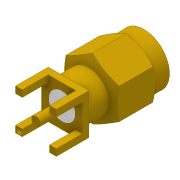
# Autodesk Inventor part: PE4525
Saved by Autodesk Inventor 2017 (Build 210142000, 142)
## iProperties
Created: 2020-05-17
Part Number: PE4525
Material: Aluminum 6061
Document SubType Name: Modeling
Designer: Flash
Density: 2.7 g/cm^3
Appearance: Gold
Author: Flash
Autodesk Inventor part; units mm, degrees
ref_plane "YZ Plane" through (0, 0, 0) normal (1, 0, 0) x (0, 1, 0)
ref_plane "XZ Plane" through (0, 0, 0) normal (0, 1, 0) x (-1, 0, 0)
ref_plane "XY Plane" through (0, 0, 0) normal (0, 0, 1) x (1, 0, 0)
sketch "Sketch1" plane through (0, 0, 0) normal (0, 1, 0) x (-1, 0, 0)
  line L0 (3.05, 3.05) -> (2.05, 3.05)
  line L1 (2.05, 3.05) -> (2.05, 2.05)
  line L2 (2.05, 2.05) -> (3.05, 2.05)
  line L3 (3.05, 2.05) -> (3.05, 3.05)
  line L4 (3.05, 3.05) -> (2.05, 2.05) construction
  line L5 (2.05, 3.05) -> (3.05, 2.05) construction
  line L6 (3.05, -3.05) -> (2.05, -3.05)
  line L7 (2.05, -3.05) -> (2.05, -2.05)
  line L8 (2.05, -2.05) -> (3.05, -2.05)
  line L9 (3.05, -2.05) -> (3.05, -3.05)
  line L10 (3.05, -3.05) -> (2.05, -2.05) construction
  line L11 (2.05, -3.05) -> (3.05, -2.05) construction
  line L12 (-2.05, -2.05) -> (-3.05, -2.05)
  line L13 (-3.05, -2.05) -> (-3.05, -3.05)
  line L14 (-3.05, -3.05) -> (-2.05, -3.05)
  line L15 (-2.05, -3.05) -> (-2.05, -2.05)
  line L16 (-2.05, -2.05) -> (-3.05, -3.05) construction
  line L17 (-3.05, -2.05) -> (-2.05, -3.05) construction
  line L18 (-2.05, 3.05) -> (-3.05, 3.05)
  line L19 (-3.05, 3.05) -> (-3.05, 2.05)
  line L20 (-3.05, 2.05) -> (-2.05, 2.05)
  line L21 (-2.05, 2.05) -> (-2.05, 3.05)
  line L22 (-2.05, 3.05) -> (-3.05, 2.05) construction
  line L23 (-3.05, 3.05) -> (-2.05, 2.05) construction
  line L24 (0, 0) -> (1.0097, 0)
  line L25 (1.0097, 0) -> (0, 0)
  line L26 (0, 0) -> (0, -1.0471)
  circle A0 centre (0, 0) radius 0.65
  point P0 (2.55, 2.55)
  point P1 (2.55, -2.55)
  point P2 (-2.55, -2.55)
  point P3 (-2.55, 2.55)
  dimension "d0" = 1
  dimension "d1" = 1
  dimension "d2" = 1
  dimension "d3" = 1
  dimension "d4" = 1
  dimension "d5" = 1
  dimension "d6" = 1
  dimension "d7" = 1
  dimension "d8" = 5.1
  dimension "d9" = 5.1
  dimension "d10" = 1.3
  constraints: 54 end point, 9 equal length, 8 midpoint, 5 horizontal, 4 perpendicular, 4 symmetric about line, 1 centre point, 1 coincident, 1 vertical
  measures "d0" distance of L2.end L1.end
  measures "d1" distance of L1.end L0.end
  measures "d2" distance of L7.end L8.end
  measures "d3" distance of L6.end L7.end
  measures "d4" distance of L14.end L13.end
  measures "d5" distance of L13.end L12.end
  measures "d6" distance of L20.end L19.end
  measures "d7" distance of L19.end L18.end
  measures "d8" distance of point (2.55, -2.55) point (2.55, 2.55)
  measures "d9" distance of point (2.55, -2.55) point (-2.55, -2.55)
  measures "d10" diameter of A0
extrude "Extrusion1" add sketch "Sketch1" along normal blind 3.9
sketch "Sketch2" plane through (0, 3.9, 0) normal (0, 1, 0) x (1, 0, 0)
  line L0 (-2.05, 3.05) -> (-3.05, 3.05) projected
  line L1 (3.05, -3.05) -> (-3.05, -3.05)
  line L2 (-3.05, -3.05) -> (-3.05, 3.05)
  line L3 (-3.05, 3.05) -> (3.05, 3.05)
  line L4 (3.05, 3.05) -> (3.05, -3.05)
  line L5 (3.05, -3.05) -> (-3.05, 3.05) construction
  line L6 (-3.05, -3.05) -> (3.05, 3.05) construction
  point P0 (0, 0)
  constraints: 12 end point, 2 midpoint, 2 parallel, 1 horizontal, 1 perpendicular
extrude "Extrusion2" add sketch "Sketch2" along normal blind 1
sketch "Sketch3" plane through (0, 4.9, 0) normal (0, 1, 0) x (1, 0, 0)
  circle A0 centre (0, 0) radius 3.05
  constraints: 1 centre point, 1 coincident
extrude "Extrusion3" add sketch "Sketch3" along normal blind 3
sketch "Sketch4" plane through (0, 7.9, 0) normal (0, 1, 0) x (1, 0, 0)
  line L0 (-4, 2.3094) -> (0, 4.6188)
  line L1 (0, 4.6188) -> (4, 2.3094)
  line L2 (4, 2.3094) -> (4, -2.3094)
  line L3 (4, -2.3094) -> (0, -4.6188)
  line L4 (0, -4.6188) -> (-4, -2.3094)
  line L5 (-4, -2.3094) -> (-4, 2.3094)
  point P0 (0, 0)
  point P1 (0, 0)
  dimension "d17" = 8
  constraints: 12 end point, 1 coincident, 13 other
  measures "d17" distance between parallel lines of L2 L5
extrude "Extrusion4" add sketch "Sketch4" along normal blind 8.3
sketch "Sketch5" plane through (0, 0, 0) normal (1, 0, 0) x (0, 1, 0)
  line L0 (0, 0) -> (-1.897, 0)
  line L1 (18.472, 3.825) -> (14.03, 3.825)
  line L2 (14.03, 3.825) -> (14.03, 5.8463)
  line L3 (14.03, 5.8463) -> (18.472, 5.8463)
  line L4 (18.472, 5.8463) -> (18.472, 3.825)
  line L5 (16.2, 4.6188) -> (16.2, 2.3094) projected
  dimension "d20" = 3.825
  dimension "d21" = 2.17
  constraints: 10 end point, 2 horizontal, 2 parallel, 1 perpendicular
  measures "d20" distance between parallel lines of L0 L1
  measures "d21" distance between parallel lines of L2 L5
revolve "Revolution1" cut sketch "Sketch5" angle 360 about axis through (0, 0, 0) along (0, -1, 0)
sketch "Sketch6" plane through (0, 0, 0) normal (1, 0, 0) x (0, 1, 0)
  line L0 (16.2, 3.825) -> (14.03, 3.825) projected
  line L1 (14.03, 3.825) -> (12.993, 5.3625)
  line L2 (12.993, 5.3625) -> (14.03, 5.3625)
  line L3 (14.03, 4.6188) -> (14.03, 2.3094) projected
  line L4 (14.03, 5.3625) -> (14.03, 3.825)
  line L5 (4.9, 3.05) -> (7.9, 3.05) projected
  line L6 (7.9, 3.05) -> (8.7476, 5.3625)
  line L7 (8.7476, 5.3625) -> (7.9, 5.3625)
  line L8 (7.9, 5.3625) -> (7.9, 3.05)
  line L9 (0, 0) -> (-1.1331, 0)
  constraints: 14 end point, 3 point on line, 2 perpendicular, 1 collinear, 1 horizontal
revolve "Revolution2" cut sketch "Sketch6" angle 360 about axis through (0, 0, 0) along (0, -1, 0)
sketch "Sketch7" plane through (0, 16.2, 0) normal (0, 1, 0) x (1, 0, 0)
  circle A0 centre (0, 0) radius 3.2
  circle A1 centre (0, 0) radius 0.5
  dimension "d24" = 6.4
  dimension "d25" = 1
  constraints: 2 centre point, 2 coincident
  measures "d24" diameter of A0
  measures "d25" diameter of A1
extrude "Extrusion5" cut sketch "Sketch7" against normal blind 3
sketch "Sketch8" plane through (0, 0, 0) normal (0, -1, 0) x (1, 0, 0)
  line L0 (-3.05, -3.05) -> (-2.05, -3.05) projected
  line L1 (-2.05, -3.05) -> (-2.05, -2.05) projected
  line L2 (-2.05, -2.05) -> (-3.05, -2.05) projected
  line L3 (-3.05, -2.05) -> (-3.05, -3.05) projected
  circle A0 centre (-2.55, -2.55) radius 0.4512
  point P0 (0, 0)
  constraints: 1 centre point
extrude "Extrusion6" cut sketch "Sketch8" against normal blind 0.5 contours A0
sketch "Sketch9" plane through (0, 13.2, 0) normal (0, 1, 0) x (1, 0, 0)
  circle A0 centre (0, 0) radius 3.2 projected
  circle A1 centre (0, 0) radius 0.65 projected
  circle A2 centre (0, 0) radius 2.7
  dimension "d30" = 5.4
  constraints: 1 centre point, 1 coincident
  measures "d30" diameter of A2
extrude "Extrusion7" cut sketch "Sketch9" against normal blind 1.8 contours A0
fillet "Fillet1" radius 0.4 1 edges at (-2.7, 13.2, 0)
fillet "Fillet2" radius 0.4 1 edges at (-0.5, 16.2, 0)
sketch "Sketch10" plane through (0, 3.9, 0) normal (0, -1, 0) x (1, 0, 0)
  circle A0 centre (0, 0) radius 0.5 projected
  circle A1 centre (0, 0) radius 2
  dimension "d35" = 4
  constraints: 1 centre point, 1 coincident
  measures "d35" diameter of A1
extrude "Extrusion8" cut sketch "Sketch10" against normal blind 0.01
body "Solid1"
